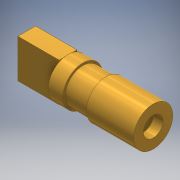
# Autodesk Inventor part: laser_taida_6mm
Saved by Autodesk Inventor 2016 (Build 200138000, 138)
## iProperties
Created: 2016-08-10
Part Number: laser_taida_6mm
Material: Brass, Soft Yellow
Document SubType Name: Modeling
Designer: rawrdong
Density: 8.47 g/cm^3
Appearance: Brass - Satin
Author: rawrdong
Autodesk Inventor part; units mm, degrees
ref_plane "YZ Plane" through (0, 0, 0) normal (1, 0, 0) x (0, 1, 0)
ref_plane "XZ Plane" through (0, 0, 0) normal (0, 1, 0) x (-1, 0, 0)
ref_plane "XY Plane" through (0, 0, 0) normal (0, 0, 1) x (1, 0, 0)
sketch "Sketch1" plane through (0, 0, 0) normal (0, 0, 1) x (1, 0, 0)
  line L0 (0, 0) -> (11.5, 0)
  line L1 (13, 1.5) -> (13, 2.99)
  line L2 (13, 2.99) -> (5.8, 2.99)
  line L3 (5.8, 2.99) -> (5.8, 2.7)
  line L4 (5.8, 2.7) -> (2.26, 2.7)
  line L5 (2.26, 2.7) -> (2.26, 3.025)
  line L6 (2.26, 3.025) -> (0, 3.025)
  line L7 (0, 3.025) -> (0, 0)
  line L8 (13, 1.5) -> (11.5, 1.5)
  line L9 (11.5, 1.5) -> (11.5, 0)
  dimension "d0" = 7.2
  dimension "d1" = 5.98
  dimension "d2" = 2.26
  dimension "d3" = 6.05
  dimension "d4" = 3
  dimension "d5" = 1.5
  dimension "d6" = 13
  dimension "d7" = 5.4
  constraints: 20 end point, 7 perpendicular, 2 horizontal
  measures "d0" distance between parallel lines of L1 L3
  measures "d1" diameter of L2 L0
  measures "d2" distance between parallel lines of L5 L7
  measures "d3" diameter of L6 L0
  measures "d4" diameter of L8 L0
  measures "d5" distance between parallel lines of L1 L9
  measures "d6" distance between parallel lines of L7 L1
  measures "d7" diameter of L4 L0
revolve "Revolution1" add sketch "Sketch1" angle 360 about axis through (0, 0, 0) along (1, 0, 0)
sketch "Sketch2" plane through (0, 0, 0) normal (-1, 0, 0) x (0, 0, 1)
  line L0 (-2.95, -1.35) -> (2.95, -1.35)
  line L1 (2.95, -1.35) -> (2.95, 1.35)
  line L2 (2.95, 1.35) -> (-2.95, 1.35)
  line L3 (-2.95, 1.35) -> (-2.95, -1.35)
  line L4 (-2.95, -1.35) -> (2.95, 1.35) construction
  line L5 (2.95, -1.35) -> (-2.95, 1.35) construction
  point P0 (0, 0)
  dimension "d9" = 5.9
  dimension "d10" = 2.7
  constraints: 12 end point, 2 midpoint, 2 parallel, 1 horizontal, 1 perpendicular
  measures "d9" distance of L1.end L2.end
  measures "d10" distance of L0.end L1.end
extrude "Extrusion1" add sketch "Sketch2" along normal blind 6.3
body "Solid1"
